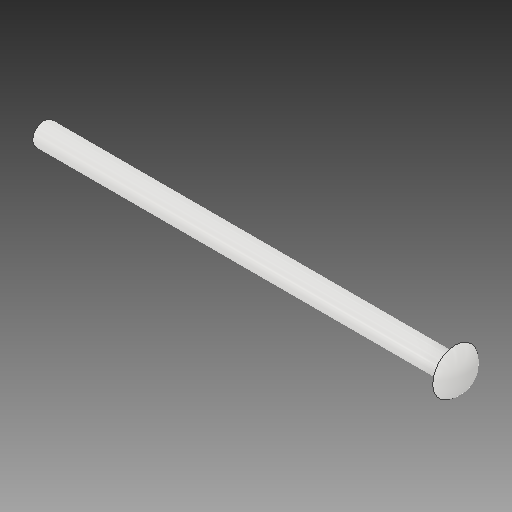
# Autodesk Inventor part: Pasador del Mango
Saved by Autodesk Inventor 2020 (Build 240168000, 168)
## iProperties
Created: 2016-05-05
Part Number: Pasador del Mango
Material: Aluminum
Document SubType Name: Modeling
Designer: Jorge
Mass: 7.11232 g
Surface Area: 19.9912 cm^2
Volume: 2.63419 cm^3
Density: 2.7 g/cm^3
Appearance: Satin
Author: Jorge
Autodesk Inventor part; units mm, degrees
ref_plane "YZ Plane" through (0, 0, 0) normal (1, 0, 0) x (0, 1, 0)
ref_plane "XZ Plane" through (0, 0, 0) normal (0, 1, 0) x (-1, 0, 0)
ref_plane "XY Plane" through (0, 0, 0) normal (0, 0, 1) x (1, 0, 0)
sketch "Sketch1" plane through (0, 0, 0) normal (0, 0, 1) x (1, 0, 0)
  line L0 (0, 2.7781) -> (101.6, 2.7781)
  arc A0 (104.775, 0) -> (101.6, 5.5563) centre (98.3258, 0) ccw
  line L1 (101.6, 2.7781) -> (101.6, 5.5563)
  line L2 (-21.1026, 0) -> (126.6153, 0) projected
  line L3 (0, -1.1956) -> (0, 7.1734) construction
  line L4 (0, 2.7781) -> (0, 0)
  line L5 (0, 0) -> (104.775, 0)
  dimension "d0" = 101.6
  dimension "d1" = 11.1125
  dimension "d2" = 3.175
  dimension "d3" = 5.5563
  constraints: 8 end point, 3 point on line, 2 point on circle, 1 centre point, 1 collinear, 1 horizontal, 1 perpendicular, 1 vertical
  measures "d0" distance between parallel lines of L3 L1
  measures "d1" diameter of L1.end L2
  measures "d2" distance from line of L5.end L1
  measures "d3" diameter of L0 L2
revolve "Revolution1" add sketch "Sketch1" angle 360 about axis through (-10, 0, 0) along (1, 0, 0)
body "Solid1"
